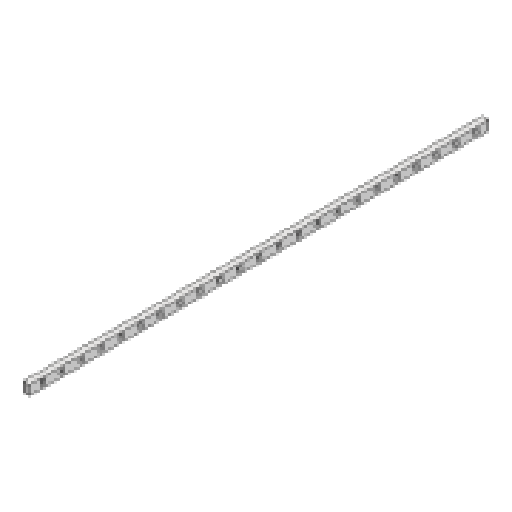
# Autodesk Inventor part: mgn7 rail
Saved by Autodesk Inventor 2023 (Build 270158000, 158)
## iProperties
Created: 2022-10-31
Part Number: mgn7 rail
Material: Generic
Document SubType Name: Modeling
Designer: deli
Density: 1 g/cm^3
Appearance: Default
Author: deli
Autodesk Inventor part; units mm, degrees
ref_plane "YZ Plane" through (0, 0, 0) normal (1, 0, 0) x (0, 1, 0)
ref_plane "XZ Plane" through (0, 0, 0) normal (0, 1, 0) x (-1, 0, 0)
ref_plane "XY Plane" through (0, 0, 0) normal (0, 0, 1) x (1, 0, 0)
sketch "Sketch1" plane through (0, 0, 0) normal (0, 0, 1) x (1, 0, 0)
  line L0 (-12.5153, 6.9424) -> (-7.7153, 6.9424)
  line L1 (-7.7153, 6.9424) -> (-7.7153, -0.0576)
  line L2 (-7.7153, -0.0576) -> (-12.5153, -0.0576)
  line L3 (-12.5153, -0.0576) -> (-12.5153, 6.9424)
  point P0 (0, 0)
  dimension "d0" = 4.8
  dimension "d1" = 7
  constraints: 8 end point, 2 parallel, 1 horizontal, 1 perpendicular
  measures "d0" distance of L0.start L0.end
  measures "d1" distance of L0.end L1.end
extrude "Extrusion1" add sketch "Sketch1" along normal blind 350
sketch "Sketch2" plane through (-7.7153, 6.9424, 350) normal (1, 0, 0) x (0, 0, -1)
  line L0 (350, -7) -> (350, 0) projected
  line L1 (350, -7) -> (0, -7) projected
  circle A0 centre (340, -3.5) radius 1.2
  circle A1 centre (325, -3.5) radius 1.2
  circle A2 centre (310, -3.5) radius 1.2
  circle A3 centre (295, -3.5) radius 1.2
  circle A4 centre (280, -3.5) radius 1.2
  circle A5 centre (265, -3.5) radius 1.2
  circle A6 centre (250, -3.5) radius 1.2
  circle A7 centre (235, -3.5) radius 1.2
  circle A8 centre (220, -3.5) radius 1.2
  circle A9 centre (205, -3.5) radius 1.2
  circle A10 centre (190, -3.5) radius 1.2
  circle A11 centre (175, -3.5) radius 1.2
  circle A12 centre (160, -3.5) radius 1.2
  circle A13 centre (145, -3.5) radius 1.2
  circle A14 centre (130, -3.5) radius 1.2
  circle A15 centre (115, -3.5) radius 1.2
  circle A16 centre (100, -3.5) radius 1.2
  circle A17 centre (85, -3.5) radius 1.2
  circle A18 centre (70, -3.5) radius 1.2
  circle A19 centre (55, -3.5) radius 1.2
  circle A20 centre (40, -3.5) radius 1.2
  circle A21 centre (25, -3.5) radius 1.2
  circle A22 centre (10, -3.5) radius 1.2
  point P0 (350, -6.9424)
  dimension "d4" = 2.4
  dimension "d5" = 3.5
  dimension "d8" = 15
  dimension "d13" = 330
  dimension "d14" = 10
  constraints: 23 centre point, 1 horizontal, 44 other
  measures "d4" diameter of A0
  measures "d5" distance from line of L1 A0.centre
  measures "d8" distance of A0.centre A1.centre
  measures "d13" distance of A22.centre A0.centre
  measures "d14" distance from line of L0 A0.centre
extrude "Extrusion2" cut sketch "Sketch2" against normal blind 10
sketch "Sketch3" plane through (-7.7153, 6.9424, 350) normal (1, 0, 0) x (0, 0, -1)
  circle A0 centre (340, -3.5) radius 1.2 construction
  circle A1 centre (340, -3.5) radius 2.1
  line L0 (350, -7) -> (0, -7) projected
  circle A2 centre (325, -3.5) radius 2.1
  circle A3 centre (310, -3.5) radius 2.1
  circle A4 centre (295, -3.5) radius 2.1
  circle A5 centre (280, -3.5) radius 2.1
  circle A6 centre (265, -3.5) radius 2.1
  circle A7 centre (250, -3.5) radius 2.1
  circle A8 centre (235, -3.5) radius 2.1
  circle A9 centre (220, -3.5) radius 2.1
  circle A10 centre (205, -3.5) radius 2.1
  circle A11 centre (190, -3.5) radius 2.1
  circle A12 centre (175, -3.5) radius 2.1
  circle A13 centre (160, -3.5) radius 2.1
  circle A14 centre (145, -3.5) radius 2.1
  circle A15 centre (130, -3.5) radius 2.1
  circle A16 centre (115, -3.5) radius 2.1
  circle A17 centre (100, -3.5) radius 2.1
  circle A18 centre (85, -3.5) radius 2.1
  circle A19 centre (70, -3.5) radius 2.1
  circle A20 centre (55, -3.5) radius 2.1
  circle A21 centre (40, -3.5) radius 2.1
  circle A22 centre (25, -3.5) radius 2.1
  circle A23 centre (10, -3.5) radius 2.1
  point P0 (350, -6.9424)
  dimension "d17" = 4.2
  dimension "d20" = 15
  constraints: 23 centre point, 1 coincident, 1 horizontal, 44 other
  measures "d17" diameter of A1
  measures "d20" distance of A1.centre A2.centre
extrude "Extrusion3" cut sketch "Sketch3" against normal blind 2.3
body "Solid1"
